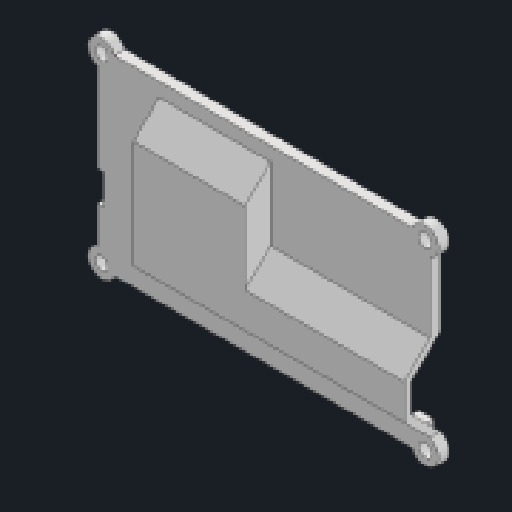
# Autodesk Inventor part: Top_case
Saved by Autodesk Inventor 2026.2 (Build 302298000, 298)
## iProperties
Created: 2026-04-11
Part Number: Top_case
Material: Generic
Document SubType Name: Modeling
Designer: Malthe Sennels
Density: 1 g/cm^3
Appearance: Default
Author: Malthe Sennels
Autodesk Inventor part; units mm, degrees
ref_plane "YZ Plane" through (0, 0, 0) normal (1, 0, 0) x (0, 1, 0)
ref_plane "XZ Plane" through (0, 0, 0) normal (0, 1, 0) x (-1, 0, 0)
ref_plane "XY Plane" through (0, 0, 0) normal (0, 0, 1) x (1, 0, 0)
sketch "Sketch1" plane through (0, 0, 0) normal (0, 0, 1) x (1, 0, 0)
  arc A0 (-46.3925, 24.0714) -> (-43.8475, 26.6164) centre (-45.0925, 25.3164) ccw
  line L0 (-46.3925, 9.0304) -> (-46.3925, 24.0714)
  line L1 (-46.3925, 9.0304) -> (-44.3931, 9.0304)
  line L2 (-44.3925, 21.1036) -> (-44.3931, 9.0304)
  arc A1 (-44.3925, 21.1036) -> (-40.8797, 24.6164) centre (-43.8925, 24.1164) ccw
  line L3 (40.9925, 24.6164) -> (-40.8797, 24.6164)
  line L4 (40.9925, 16.6164) -> (40.9925, 24.6164)
  line L5 (44.3925, 16.6164) -> (40.9925, 16.6164)
  line L6 (44.3925, 2.4144) -> (44.3925, 16.6164)
  line L7 (44.3925, 2.4144) -> (46.3925, 2.4144)
  line L8 (46.3925, 24.0714) -> (46.3925, 2.4144)
  arc A2 (43.8475, 26.6164) -> (46.3925, 24.0714) centre (45.0925, 25.3164) ccw
  line L9 (-43.8475, 26.6164) -> (43.8475, 26.6164)
  arc A3 (-43.8475, -26.6164) -> (-46.3925, -24.0714) centre (-45.0925, -25.3164) ccw
  line L10 (43.8475, -26.6164) -> (-43.8475, -26.6164)
  arc A4 (46.3925, -24.0714) -> (43.8475, -26.6164) centre (45.0925, -25.3164) ccw
  line L11 (46.3925, -21.5856) -> (46.3925, -24.0714)
  line L12 (46.3925, -21.5856) -> (44.3925, -21.5856)
  line L13 (44.3925, -19.6418) -> (44.3925, -21.5856)
  line L14 (40.3925, -19.6418) -> (44.3925, -19.6418)
  line L15 (40.3925, -24.6418) -> (40.3925, -19.6418)
  line L16 (-40.8818, -24.6418) -> (40.3925, -24.6418)
  arc A5 (-40.8818, -24.6418) -> (-42.6446, -21.3551) centre (-43.8945, -24.1416) ccw
  line L17 (-46.3925, -21.3551) -> (-42.6446, -21.3551)
  line L18 (-46.3925, -24.0714) -> (-46.3925, -21.3551)
  line L19 (-46.3925, -21.7457) -> (-46.3925, -24.0714)
  arc A6 (-46.3925, -21.7457) -> (-41.5218, -26.6164) centre (-45.0925, -25.3164) ccw
  line L20 (-43.8475, -26.6164) -> (-41.5218, -26.6164)
  arc A7 (-46.3925, -24.0714) -> (-43.8475, -26.6164) centre (-45.0925, -25.3164) ccw
  line L21 (41.5218, -26.6164) -> (43.8475, -26.6164)
  arc A8 (41.5218, -26.6164) -> (46.3925, -21.7457) centre (45.0925, -25.3164) ccw
  line L22 (46.3925, -24.0714) -> (46.3925, -21.7457)
  arc A9 (43.8475, -26.6164) -> (46.3925, -24.0714) centre (45.0925, -25.3164) ccw
  line L23 (46.3925, 21.7457) -> (46.3925, 24.0714)
  arc A10 (46.3925, 21.7457) -> (41.5218, 26.6164) centre (45.0925, 25.3164) ccw
  line L24 (43.8475, 26.6164) -> (41.5218, 26.6164)
  arc A11 (46.3925, 24.0714) -> (43.8475, 26.6164) centre (45.0925, 25.3164) ccw
  line L25 (-41.5218, 26.6164) -> (-43.8475, 26.6164)
  arc A12 (-41.5218, 26.6164) -> (-46.3925, 21.7457) centre (-45.0925, 25.3164) ccw
  line L26 (-46.3925, 24.0714) -> (-46.3925, 21.7457)
  arc A13 (-43.8475, 26.6164) -> (-46.3925, 24.0714) centre (-45.0925, 25.3164) ccw
  line L27 (44.3925, 2.4144) -> (0, 2.4144)
  line L28 (0, 2.4144) -> (0, 24.6164)
  line L29 (44.3925, -21.5856) -> (0, -21.5856)
  line L30 (-44.3937, -2.9696) -> (-46.3925, -2.9696)
  line L31 (-46.3925, -11.5551) -> (-46.3925, -2.9696)
  line L32 (-44.3941, -11.5551) -> (-46.3925, -11.5551)
  line L33 (-44.3937, -2.9696) -> (-44.3941, -11.5551)
  line L34 (-46.3925, -21.7457) -> (-46.3925, -11.5551)
  line L35 (-46.3925, -2.9696) -> (-46.3925, 9.0304)
  line L36 (0, -11.3836) -> (-27, -11.3836)
  line L37 (-27, -11.3836) -> (-27, 15.6164)
  line L38 (-27, 15.6164) -> (0, 15.6164)
  line L39 (0, 15.6164) -> (0, -11.3836)
  line L40 (0, -11.3836) -> (0, -21.5856)
  point P0 (0, 0)
  point P1 (40.3925, -21.5856)
  point P2 (0, 15.6164)
extrude "Extrusion1" add sketch "Sketch1" along normal blind 3 contours A0 L9 A2 L8 L7 L6 L5 L4 L3 A1 L2 L1 L0 | L0 A12 L9 A13 | L1 L2 A1 L3 L28 L38 L37 L36 L40 L29 L15 L16 A5 L17 L34 L32 L33 L30 L35 | A10 L8 A11 L9 | L17 A5 L16 L15 L29 L12 L11 A4 L10 A3 L18 | L27 L28 L3 L4 L5 L6 | L18 A7 L10 A6 | L10 A9 L11 A8 | L15 L14 L13 L29
sketch "Sketch2" plane through (44.3925, -21.5856, 0) normal (1, 0, 0) x (0, 0, -1)
  line L0 (0, 0) -> (-8, 8) projected
  line L1 (-8, 16) -> (0, 24) projected
  line L2 (-8, 8) -> (-8, 16) projected
  line L3 (-0.0707, -0.0707) -> (-8.1, 7.9586)
  line L4 (-8.1, 7.9586) -> (-8.1, 16.0414)
  line L5 (-8.1, 16.0414) -> (-0.0707, 24.0707)
  line L6 (0, 0) -> (-3, 0) projected
  line L7 (0, 24) -> (-3, 24) projected
  line L8 (-3, 0) -> (-10.1, 7.1)
  line L9 (-10.1, 7.1) -> (-10.1, 16.9)
  line L10 (-10.1, 16.9) -> (-3, 24)
  point P0 (0, 21.5856)
  point P1 (-0.1414, 24)
  point P2 (-0.1414, 0)
  dimension "d5" = 0.1
  dimension "d6" = 2
  constraints: 12 end point, 1 parallel, 1 perpendicular, 1 vertical, 2 other
  measures "d5" distance between parallel lines of L0 L3
  measures "d6" distance between parallel lines of L4 L9
extrude "Extrusion2" add sketch "Sketch2" along normal blind 2 and the other way blind 71.5 contours L6 L8 L9 L10 L7 L5 L4 L3
sketch "Sketch3" plane through (0, 0, 3) normal (0, 0, 1) x (1, 0, 0)
  line L0 (0, 15.6164) -> (0, 2.4144) projected
  line L1 (-27.1075, -21.5856) -> (-27.1075, -14.4856) projected
  line L2 (0, 15.6164) -> (-27.1075, 15.6164)
  line L3 (-27.1075, 15.6164) -> (-27.1075, -14.4856)
  line L4 (-27.1075, -14.4856) -> (0, -14.4856)
  line L5 (0, -14.4856) -> (0, 15.6164)
  point P0 (0, 0)
  point P1 (0, 2.4144)
  constraints: 8 end point, 2 parallel, 1 horizontal, 1 perpendicular
extrude "Extrusion3" cut sketch "Sketch3" along normal blind 10 and the other way blind 3.25
sketch "Sketch4" plane through (0, 2.4144, 0) normal (-1, 0, 0) x (0, 0, 1)
  line L0 (10.1, -16.9) -> (7.2414, -16.9) projected
  line L1 (8.1, -16.0414) -> (8.1, -7.9586) projected
  line L2 (8.1, -15.8474) -> (8.1, -16.9)
  line L3 (8.1, -16.9) -> (10.1, -16.9)
  line L4 (10.1, -16.9) -> (10.1, 13.202)
  line L5 (10.1, 13.202) -> (8.1, 13.202)
  line L6 (8.1, 13.202) -> (8.1, -16.9)
  line L7 (10.1, 13.202) -> (2.1168, 21.1852)
  line L8 (10.1, 13.202) -> (21.3899, 13.202) construction
  line L9 (3, 13.202) -> (3, 0) projected
  line L10 (3, 0) -> (3, 19.3313) projected
  line L11 (3, 19.3313) -> (3, 24.202) projected
  line L12 (3, 24.202) -> (3, 19.3313) projected
  line L13 (3, 19.3313) -> (3, -5.384) projected
  line L14 (3, -5.384) -> (3, -13.9695) projected
  line L15 (3, -13.9695) -> (3, -24.1601) projected
  line L16 (3, -24.1601) -> (3, -29.0308) projected
  line L17 (3, -29.0308) -> (3, -24.1601) projected
  line L18 (3, -24.1601) -> (3, -24) projected
  line L19 (3, -24) -> (3, -21.1414) projected
  line L20 (3, -21.1414) -> (3, -16.9) projected
  line L21 (3, -16.9) -> (3, 13.202) projected
  line L22 (3, 24.702) -> (3, 21.102) projected
  line L23 (3, -25.9308) -> (3, -29.5308) projected
  line L24 (3, -25.9308) -> (3, -29.5308) projected
  line L25 (3, 24.702) -> (3, 21.102) projected
  line L26 (8.1, 13.202) -> (3, 18.302)
  point P0 (0, -2.4144)
  point P1 (10.1, -7.1)
  point P2 (8.1, -7.9586)
  point P3 (3, 20.302)
  point P4 (3, 18.302)
  dimension "d15" = 135
  constraints: 16 end point, 5 point on line, 3 parallel, 2 horizontal, 2 perpendicular, 1 equal length
  measures "d15" angle of L8 L7
extrude "Extrusion4" add sketch "Sketch4" along normal up to surface (27.1075 mm away)
sketch "Sketch5" plane through (0, 2.4144, 0) normal (1, 0, 0) x (0, 0, -1)
  line L0 (-10.1, -7.1) -> (-10.1, 13.202) projected
  line L1 (-8.1, -5.1) -> (-10.1, -7.1) projected
  line L2 (-8.1, 13.202) -> (-8.1, -5.1) projected
  line L3 (-3, 18.302) -> (-8.1, 13.202) projected
  line L4 (-3, 20.302) -> (-3, 18.302) projected
  line L5 (-10.1, 13.202) -> (-3, 20.302) projected
  line L6 (-10.1, -7.1) -> (-10.1, 13.202) projected
  line L7 (-3, 18.302) -> (-3, 0)
  line L8 (-3, 0) -> (-8.1, -5.1)
  point P0 (0, -2.4144)
  point P1 (-10.1, 13.202)
  constraints: 4 end point
extrude "Extrusion5" add sketch "Sketch5" along normal blind 2
sketch "Sketch6" plane through (-27.1075, -21.5856, 0) normal (-1, 0, 0) x (0, 0, 1)
  line L0 (8.1, 7.1) -> (7.2414, 7.1) projected
  line L1 (7.2414, 7.1) -> (3, 2.8586) projected
  line L2 (3, 0) -> (3, 2.8586) projected
  line L3 (3, 0) -> (10.1, 7.1) projected
  line L4 (10.1, 37.202) -> (10.1, 7.1) projected
  line L5 (3, 44.302) -> (10.1, 37.202) projected
  line L6 (3, 42.302) -> (3, 44.302) projected
  line L7 (8.1, 37.202) -> (3, 42.302) projected
  line L8 (8.1, 7.1) -> (8.1, 37.202) projected
  line L9 (3, 0) -> (14.0396, 0)
  line L10 (14.0396, 0) -> (14.0396, 45.0941)
  line L11 (14.0396, 45.0941) -> (3, 45.0941)
  line L12 (3, 45.0941) -> (3, 0)
  point P0 (0, 21.5856)
  point P1 (3, 2.8586)
  constraints: 8 end point, 2 parallel, 1 horizontal, 1 perpendicular
extrude "Extrusion6" add sketch "Sketch6" along normal blind 2 contours L8 L7 L6 L5 L4 L3 L2 L1 L0 | L0 L1 L12 L7 L8
sketch "Sketch7" plane through (0, -21.5856, 0) normal (1, 0, 0) x (0, 0, -1)
  line L0 (0, 7.1) -> (-3, 7.1) projected
  line L1 (-3, 2.8586) -> (-3, 7.1) projected
  line L2 (-3, 2.8586) -> (-0.1414, 0) projected
  line L3 (0, 0) -> (-0.1414, 0) projected
  line L4 (0, 0) -> (0, 7.1) projected
  point P0 (0, 21.5856)
extrude "Extrusion7" cut sketch "Sketch7" against normal up to surface (27.1075 mm away)
sketch "Sketch8" plane through (0, 0, 3) normal (0, 0, 1) x (1, 0, 0)
  line L0 (35.1595, -0.5396) -> (31.9595, -0.5396)
  line L1 (31.9595, -0.5396) -> (31.9595, 14.6261)
  line L2 (31.9595, 14.6261) -> (35.1595, 14.6261)
  line L3 (35.1595, 14.6261) -> (35.1595, -0.5396)
  line L4 (34.1345, -0.0368) -> (34.1345, -0.9368) projected
  line L5 (32.9845, -0.0368) -> (32.9845, -0.9368) projected
  line L6 (32.9845, -0.7101) -> (34.1345, -0.7101)
  line L7 (33.5595, -0.7101) -> (33.5595, 14.6138)
  point P0 (0, 0)
  dimension "d24" = 3.2
  dimension "d25" = 1.6
  constraints: 12 end point, 3 perpendicular, 2 parallel, 2 point on line, 1 horizontal, 1 midpoint
  measures "d24" distance of L1.end L2.end
  measures "d25" distance from line of L7.end L3
extrude "Extrusion8" cut sketch "Sketch8" along normal blind 10 and the other way blind 5 contours L0 L1 L2 L3
sketch "Sketch9" plane through (-46.3925, -2.9696, 0) normal (-1, 0, 0) x (0, 0, 1)
  line L0 (-6.415, 12) -> (0, 12) projected
  line L1 (3, 0) -> (-6.415, 0) projected
  line L2 (-6.415, 11.8) -> (0, 11.8)
  line L3 (3, 0.2) -> (-6.415, 0.2)
  line L4 (0, 5.384) -> (0, 24.7153) projected
  arc A0 (0, 9.8) -> (-2, 11.8) centre (-2, 9.8) ccw
  line L5 (0, 24.7153) -> (0, 0) projected
  arc A1 (-1.8751, 0.2) -> (0, 2.0751) centre (-1.8751, 2.0751) ccw
  point P0 (0, 2.9696)
  dimension "d30" = 0.2
  dimension "d31" = 0.2
  dimension "d32" = 2
  constraints: 4 end point, 4 point on circle, 4 point on line, 4 tangent, 2 centre point, 2 parallel
  measures "d30" distance between parallel lines of L0 L2
  measures "d31" distance between parallel lines of L1 L3
  measures "d32" radius of A0
body "Solid1"
